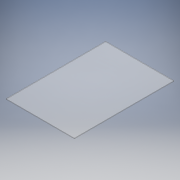
# Autodesk Inventor part: Plaque coté
Saved by Autodesk Inventor 2017 (Build 210142000, 142)
## iProperties
Company: FABLAB Frenchmakers
Part Number: Plaque coté
Project: 1400-PopCorn Machine
Material: Plastique PMMA
Catalog Web Link: http://www.frenchmakers.com/
Document SubType Name: Modeling
Designer: FABLAB Frenchmakers
Density: 1.188 g/cm^3
Appearance: Polycarbonate - Transparent
Stock Number: 1400-04-03
Author: Adrien MARY
Autodesk Inventor part; units mm, degrees
ref_plane "YZ Plane" through (0, 0, 0) normal (1, 0, 0) x (0, 1, 0)
ref_plane "XZ Plane" through (0, 0, 0) normal (0, 1, 0) x (-1, 0, 0)
ref_plane "XY Plane" through (0, 0, 0) normal (0, 0, 1) x (1, 0, 0)
sketch "Esquisse1" plane through (0, 0, 0) normal (0, 0, 1) x (1, 0, 0)
  line L0 (-153.7, -224) -> (153.7, -224)
  line L1 (153.7, -224) -> (153.7, 224)
  line L2 (153.7, 224) -> (-153.7, 224)
  line L3 (-153.7, 224) -> (-153.7, -224)
  line L4 (-153.7, -224) -> (153.7, 224) construction
  line L5 (153.7, -224) -> (-153.7, 224) construction
  point P0 (0, 0)
  dimension "Profondeur_plaque_coté" = 307.4
  dimension "Hauteur_plaque_coté" = 448
  constraints: 12 end point, 2 midpoint, 2 parallel, 1 horizontal, 1 perpendicular
  measures "Profondeur_plaque_coté" distance of L2.end L1.end
  measures "Hauteur_plaque_coté" distance of L0.end L1.end
extrude "Embase" add sketch "Esquisse1" along normal mid plane 3
